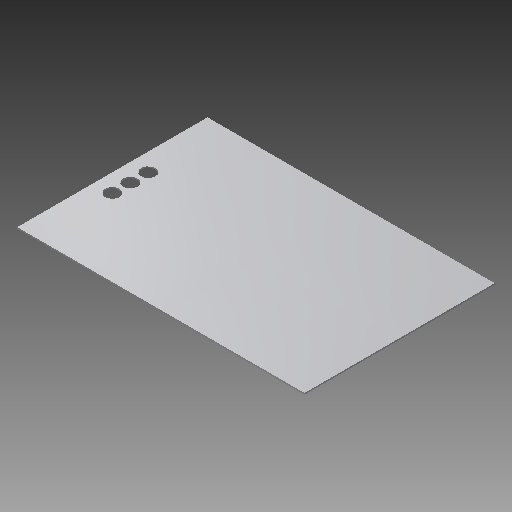
# Autodesk Inventor part: Käfigboden
Saved by Autodesk Inventor 2018 (Build 220112000, 112)
## iProperties
Created: 2012-11-27
Part Number: Käfigboden
Material: PVC-U
Document SubType Name: Modeling
Designer: Neef
Mass: 2373.5 g
Surface Area: 8583.18 cm^2
Volume: 1695.36 cm^3
Density: 1.4 g/cm^3
Appearance: Smooth - White
Author: Neef
Autodesk Inventor part; units mm, degrees
ref_plane "YZ Plane" through (0, 0, 0) normal (1, 0, 0) x (0, 1, 0)
ref_plane "XZ Plane" through (0, 0, 0) normal (0, 1, 0) x (-1, 0, 0)
ref_plane "XY Plane" through (0, 0, 0) normal (0, 0, 1) x (1, 0, 0)
sketch "Skizze1" plane through (0, 0, 0) normal (0, 0, 1) x (1, 0, 0)
  line L0 (0, 370.86) -> (0, -370.86) projected
  line L1 (-560, 0) -> (560, 0) projected
  line L2 (400, -264.9) -> (-400, -264.9)
  line L3 (-400, -264.9) -> (-400, 264.9)
  line L4 (-400, 264.9) -> (400, 264.9)
  line L5 (400, 264.9) -> (400, -264.9)
  point P0 (0, 0)
  point P1 (0, -264.9)
  point P2 (-400, 0)
  dimension "d0" = 800
  dimension "d1" = 529.8
  constraints: 8 end point, 2 midpoint, 2 parallel, 2 point on line, 1 horizontal, 1 perpendicular
  measures "d0" distance of L2.start L2.end
  measures "d1" distance of L2.end L3.end
extrude "Extrusion1" add sketch "Skizze1" along normal blind 4
sketch "Skizze2" plane through (0, 0, 0) normal (0, 0, -1) x (-1, 0, 0)
  line L0 (400, 264.9) -> (400, -264.9) projected
  line L1 (-400, 264.9) -> (400, 264.9) projected
  point P0 (0, 0)
  point P1 (350, 50)
  point P2 (350, 0)
  point P3 (350, -50)
  dimension "d4" = 50
  dimension "d5" = 50
  dimension "d6" = 50
  dimension "d7" = 50
  dimension "d8" = 50
  dimension "d9" = 264.9
  measures "d4" distance from line of L0 point (350, 50)
  measures "d5" distance from line of L0 point (350, 0)
  measures "d6" distance from line of L0 point (350, -50)
  measures "d7" distance of point (350, 0) point (350, 50)
  measures "d8" distance of point (350, 0) point (350, -50)
  measures "d9" distance from line of L1 point (350, 0)
hole "Bohrung1" at (-350, 50, 0) at (-350, 0, 0) at (-350, -50, 0) direction (0, 0, 1) diameter 40 end through all
equation "\"d5\" = d4"
equation "\"d6\" = d5"
equation "\"d8\" = d7"
